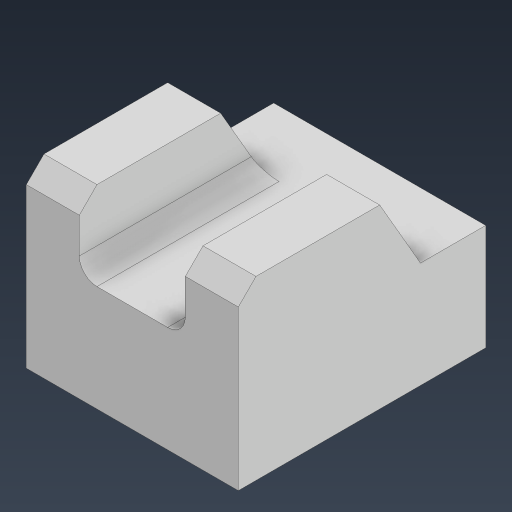
# Autodesk Inventor part: 3D Model
Saved by Autodesk Inventor 2024 (Build 280153000, 153)
## iProperties
Created: 2024-03-05
Part Number: 3D Model
Material: Genérico
Document SubType Name: Modeling
Designer: Administrator
Density: 1 g/cm^3
Appearance: Padrão
Author: Administrator
Autodesk Inventor part; units mm, degrees
ref_plane "YZ Plane" through (0, 0, 0) normal (1, 0, 0) x (0, 1, 0)
ref_plane "XZ Plane" through (0, 0, 0) normal (0, 1, 0) x (-1, 0, 0)
ref_plane "XY Plane" through (0, 0, 0) normal (0, 0, 1) x (1, 0, 0)
sketch "Esboço1" plane through (0, 0, 0) normal (0, 1, 0) x (-1, 0, 0)
  line L0 (30, -35) -> (-30, -35)
  line L1 (-30, -35) -> (-30, 35)
  line L2 (-30, 35) -> (30, 35)
  line L3 (30, 35) -> (30, -35)
  line L4 (30, -35) -> (-30, 35) construction
  line L5 (-30, -35) -> (30, 35) construction
  point P0 (0, 0)
  dimension "d0" = 60
  dimension "d1" = 70
  constraints: 12 end point, 2 midpoint, 2 parallel, 1 horizontal, 1 perpendicular
  measures "d0" distance of L1.end L2.end
  measures "d1" distance of L0.end L1.end
extrude "Extrusão1" add sketch "Esboço1" along normal blind 50
sketch "Esboço3" plane through (30, 0, 35) normal (1, 0, 0) x (0, 0, -1)
  line L0 (0, 50) -> (70, 50) projected
  line L1 (40, 50) -> (51.547, 30)
  line L2 (51.547, 30) -> (70, 30)
  line L3 (40, 50) -> (70, 50)
  line L4 (70, 0) -> (70, 50) projected
  line L5 (70, 30) -> (70, 50)
  point P0 (35, 0)
  dimension "d6" = 20
  dimension "d7" = 30
  dimension "d8" = 60
  constraints: 8 end point, 2 collinear, 1 parallel, 1 point on line
  measures "d6" distance between parallel lines of L0 L2
  measures "d7" distance of L0.end L1.start
  measures "d8" angle of L1 L0
extrude "Extrusão2" cut sketch "Esboço3" against normal through all
sketch "Esboço4" plane through (-30, 0, 35) normal (0, 0, 1) x (1, 0, 0)
  line L0 (15, 50) -> (45, 50)
  line L1 (45, 50) -> (45, 30)
  line L2 (45, 30) -> (15, 30)
  line L3 (15, 30) -> (15, 50)
  line L4 (0, 50) -> (60, 50) projected
  point P0 (30, 0)
  point P1 (30, 50)
  dimension "d11" = 30
  dimension "d12" = 20
  constraints: 8 end point, 2 midpoint, 2 parallel, 1 horizontal, 1 perpendicular
  measures "d11" distance of L1.end L2.end
  measures "d12" distance of L0.end L1.end
extrude "Extrusão3" cut sketch "Esboço4" against normal through all
fillet "Arredondamento1" radius 5 2 edges at (-15, 30, 9.2265) (15, 30, 9.2265)
chamfer "Chanfro1" distance 5 angle 45 2 edges at (-22.5, 50, 35) (22.5, 50, 35)
